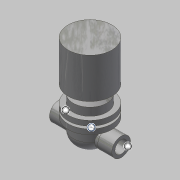
# Autodesk Inventor part: MANUEL BUTTWELD DIAFRAGM VALVE DN40
Saved by Autodesk Inventor 2017 (Build 210142000, 142)
## iProperties
Category: Piping Part
Company: Demarec
Created: 2012-12-20
Part Number: MANUEL BUTTWELD DIAFRAGM VALVE DN40
Material: 304L
Document SubType Name: Modeling
Designer: Marc Crauwels
Density: 8 g/cm^3
Mass: 658107 g
Surface Area: 21375.3 cm^2
Volume: 83622.3 cm^3
Appearance: Steel
Catalog Web Link: http://www.pocketbrewery.com
Author: Marc Crauwels
Title: Carbon Steel Globe Valve PN16
Comments: iPart CS GlbVlvPN16
Autodesk Inventor part; units mm, degrees
ref_plane "YZ Plane" through (0, 0, 0) normal (1, 0, 0) x (0, 1, 0)
ref_plane "XZ Plane" through (0, 0, 0) normal (0, 1, 0) x (-1, 0, 0)
ref_plane "XY Plane" through (0, 0, 0) normal (0, 0, 1) x (1, 0, 0)
sketch "Sketch1" plane through (0, 0, 0) normal (1, 0, 0) x (0, 1, 0)
  line L0 (84, 20) -> (98, 20)
  line L1 (98, 20) -> (98, 75)
  line L2 (98, 75) -> (84, 75)
  line L3 (84, 75) -> (84, 20)
  line L4 (98, 20) -> (100, 20)
  line L5 (100, 20) -> (100, 41)
  line L6 (100, 41) -> (98, 41)
  line L7 (98, 41) -> (98, 20)
  line L8 (-100, 0) -> (100, 0) construction
  line L9 (100, 0) -> (84, 0) construction
  line L10 (0, 0) -> (0, 254) construction
  line L11 (-100, 0) -> (-84, 0) construction
  line L12 (0, 0) -> (-10, 0)
  line L13 (-10, 0) -> (-10, 254)
  line L14 (-10, 254) -> (0, 254)
  line L15 (0, 254) -> (0, 0)
  line L16 (0, 0) -> (0, -38)
  line L17 (54, 0) -> (54, 33)
  line L18 (54, 33) -> (70, 33)
  line L19 (70, 33) -> (70, 49)
  line L20 (70, 49) -> (54, 49)
  line L21 (54, 49) -> (54, 57)
  line L22 (54, 57) -> (70, 57)
  line L23 (70, 57) -> (70, 73)
  line L24 (70, 73) -> (54, 73)
  line L25 (54, 73) -> (54, 98.4)
  line L26 (54, 98.4) -> (0, 152.4)
  line L27 (0, 152.4) -> (0, 0)
  line L28 (0, -38) -> (16, -38)
  arc A0 (16, -38) -> (54, 0) centre (16, 0) ccw
  line L29 (98, 41) -> (70, 41) construction
  line L30 (0, 125.4) -> (-70, 125.4)
  line L31 (-70, 125.4) -> (-70, 254)
  line L32 (-70, 254) -> (0, 254)
  line L33 (0, 254) -> (0, 125.4)
  point P0 (27, 125.4)
  dimension "Lenght" = 200
  dimension "DN" = 40
  dimension "FlgDia" = 150
  dimension "FlgThck" = 16
  dimension "GsktFace" = 82
  dimension "d48" = 10
  dimension "Face" = 2
  dimension "d79" = 254
  dimension "d101" = 16
  dimension "d102" = 8
  dimension "d104" = 140
  dimension "d105" = 45
  dimension "d108" = 152.4
  dimension "d112" = 70
  constraints: 68 end point, 13 perpendicular, 13 point on line, 8 parallel, 5 horizontal, 4 collinear, 4 equal length, 3 midpoint, 2 coincident, 2 point on circle, 2 tangent, 2 vertical, 1 centre point
  measures "Lenght" distance of L8.start L8.end
  measures "DN" diameter of L0 L8
  measures "FlgDia" diameter of L2 L8
  measures "FlgThck" distance between parallel lines of L3 L5
  measures "GsktFace" diameter of L5.end L8
  measures "d48" distance of L13.end L14.end
  measures "Face" distance of L5.end L6.end
  measures "d79" distance of L12.end L13.end
  measures "d101" distance of L18.end L19.end
  measures "d102" distance of L20.end L21.end
  measures "d104" diameter of L19 L27
  measures "d105" angle of L27 L26
  measures "d108" distance from line of L26.end L12
  measures "d112" distance between parallel lines of L31 L10
revolve "Revolution1" add sketch "Sketch1" angle 360 about axis through (0, -100, 0) along (0, 1, 0) contours L3 L2 L1 L0 | L1 L6 L5 L4
sketch "Sketch14" plane through (0, 84, 0) normal (0, -1, 0) x (-1, 0, 0)
  circle A0 centre (0, 0) radius 20 projected
  circle A1 centre (0, 0) radius 30
  dimension "d54" = 10
  dimension "d84" = 60
  constraints: 1 centre point
  measures "d54" radial gap between concentric circles of A1 A0
  measures "d84" diameter of A1
sketch "Sketch20" plane through (0, 0, 0) normal (1, 0, 0) x (0, 1, 0)
  line L0 (84, 30) -> (84, -30)
  line L1 (84, 0) -> (55, 0)
  arc A0 (0, 55) -> (55, 0) centre (55, 55) ccw
  line L2 (0, 55) -> (0, 60)
  line L3 (84, 30) -> (84, -30) projected
  line L4 (0, -96.4) -> (0, 312.4) projected
  point P0 (0, 0)
  dimension "d80" = 25
  dimension "d81" = 5
  constraints: 6 end point, 2 point on circle, 2 tangent, 1 centre point, 1 collinear, 1 horizontal, 1 midpoint, 1 perpendicular, 1 point on line
  measures "d80" vertical distance of L0.start L2.start
  measures "d81" distance of L2.start L2.end
sweep "Sweep4" add profiles "Sketch14" path "Sketch20" path curves L1 A0 L2
mirror "Mirror2" about plane through (0, 0, 0) normal (0, 1, 0) of "Revolution1", "Sweep4"
revolve "Revolution3" add sketch "Sketch1" angle 360 about axis through (0, 0, 0) along (0, 0, 1) contours L12 L13 L30 L15 | L15 L26 L25 L24 L23 L22 L21 L20 L19 L18 L17 A0 L28 L16 | L30 L13 L14 L15 | L30 L31 L32 L13
sketch "Sketch25" plane through (0, 100, 0) normal (0, 1, 0) x (1, 0, 0)
  circle A0 centre (0, 0) radius 30 projected
  circle A1 centre (0, 0) radius 75 projected
extrude "Extrusion11" cut sketch "Sketch25" against normal up to surface (16 mm away)
mirror "Mirror3" about plane through (0, 0, 0) normal (0, 1, 0) of "Extrusion11"
equation "\"Height\" = 254"
body "Solid1"
